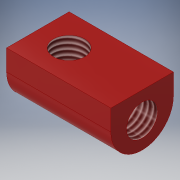
# Autodesk Inventor part: Pivot Block
Saved by Autodesk Inventor 2017 (Build 210142000, 142)
## iProperties
Created: 2017-01-12
Part Number: Pivot Block
Material: Generic
Document SubType Name: Modeling
Designer: Ben
Density: 1 g/cm^3
Appearance: Red
Author: Ben
Autodesk Inventor part; units mm, degrees
ref_plane "YZ Plane" through (0, 0, 0) normal (1, 0, 0) x (0, 1, 0)
ref_plane "XZ Plane" through (0, 0, 0) normal (0, 1, 0) x (-1, 0, 0)
ref_plane "XY Plane" through (0, 0, 0) normal (0, 0, 1) x (1, 0, 0)
sketch "Sketch1" plane through (0, 0, 0) normal (0, 1, 0) x (-1, 0, 0)
  line L0 (0, 0) -> (-31.75, 0)
  line L1 (-31.75, 0) -> (-31.75, -19.05)
  line L2 (-31.75, -19.05) -> (0, -19.05)
  line L3 (0, -19.05) -> (0, 0)
  circle A0 centre (-9.525, -9.525) radius 4.7625
  dimension "d0" = 9.525
  dimension "d1" = 19.05
  dimension "d2" = 9.525
  dimension "d3" = 9.525
  dimension "d4" = 31.75
  constraints: 8 end point, 2 parallel, 1 centre point, 1 horizontal, 1 perpendicular
  measures "d0" diameter of A0
  measures "d1" distance of L2.end L0.start
  measures "d2" distance from line of L0 A0.centre
  measures "d3" distance from line of L3 A0.centre
  measures "d4" distance of L1.end L2.end
extrude "Extrusion1" add sketch "Sketch1" along normal blind 15.875
sketch "Sketch2" plane through (31.75, 0, 0) normal (1, 0, 0) x (0, 0, -1)
  circle A0 centre (9.525, 7.9375) radius 4.7625
  line L0 (0, 0) -> (0, 15.875) projected
  line L1 (0, 0) -> (19.05, 0) projected
  dimension "d7" = 9.525
  dimension "d8" = 9.525
  dimension "d9" = 7.9375
  constraints: 1 centre point
  measures "d7" diameter of A0
  measures "d8" distance from line of L0 A0.centre
  measures "d9" distance from line of L1 A0.centre
extrude "Extrusion2" cut sketch "Sketch2" against normal blind 15.875
thread "Thread1" size "3/8-16 UNC" class "2B" standard "ANSI Unified Screw Threads" full length
thread "Thread2" size "3/8-16 UNC" class "2B" standard "ANSI Unified Screw Threads" full length
fillet "Fillet1" radius 9.525 2 edges at (15.875, 0, 0) (15.875, 0, -19.05)
body "Solid1"
